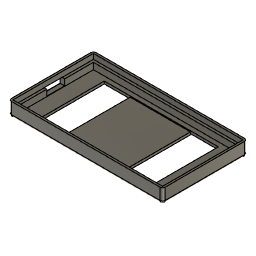
Caixa Sensores - Tampa (Autodesk Fusion 360 design; units mm, degrees)
Autodesk Fusion 360 part; units mm, degrees
note: some values were not read from the file. Set by a fixed rule: which face or edge a step refers to.
sketch "Esboço1" plane through (0, 0, 0) normal (0, 0, 1) x (1, 0, 0)
  line L0 (30, -16.5) -> (-30, -16.5)
  line L1 (-30, -16.5) -> (-30, 16.5)
  line L2 (-30, 16.5) -> (30, 16.5)
  line L3 (30, 16.5) -> (30, -16.5)
  line L4 (30, -16.5) -> (-30, 16.5) construction
  line L5 (-30, -16.5) -> (30, 16.5) construction
  dimension "d1" = 60
  dimension "d2" = 33
  constraint horizontal L0
  constraint perpendicular L0 L1
  constraint parallel L0 L2
  constraint parallel L1 L3
  constraint coincident L4 origin
  constraint coincident L5 origin
  measures "d1" distance of L1.end L2.end
  measures "d2" distance of L0.end L1.end
extrude "Extrusão1" add sketch "Esboço1" along normal blind 5.5
shell "Casca1" thickness 1.4 removed faces 1 at (10, 5.5, 5.5)
extrude "Extrusão2" add 1 faces at (28.6, -5.0333, 4.1333) along direction (-1, 0, 0) blind 0.4
extrude "Extrusão3" add 1 faces at (-9.6667, 15.1, 2.7667) along direction (0, -1, 0) blind 0.4
extrude "Extrusão4" add 1 faces at (-28.6, -5.1667, 4.1333) along direction (1, 0, 0) blind 0.4
extrude "Extrusão5" add 1 faces at (9.4, -15.1, 4.1333) along direction (0, 1, 0) blind 0.4
sketch "Esboço3" plane through (0, 0, 5.5) normal (0, 0, 1) x (-1, 0, 0)
  line L0 (-28.2, 14.7) -> (28.2, 14.7)
  line L1 (28.2, 14.7) -> (28.2, -14.7)
  line L2 (28.2, -14.7) -> (-28.2, -14.7)
  line L3 (-28.2, -14.7) -> (-28.2, 14.7)
  line L4 (-30, -16.5) -> (30, -16.5)
  line L5 (30, -16.5) -> (30, 16.5)
  line L6 (30, 16.5) -> (-30, 16.5)
  line L7 (-30, 16.5) -> (-30, -16.5)
  line L8 (29.2, -15.7) -> (-29.2, -15.7)
  line L9 (-29.2, -15.7) -> (-29.2, 15.7)
  line L10 (-29.2, 15.7) -> (29.2, 15.7)
  line L11 (29.2, 15.7) -> (29.2, -15.7)
  line L12 (29.2, -15.7) -> (-29.2, 15.7) construction
  line L13 (-29.2, -15.7) -> (29.2, 15.7) construction
  dimension "d16" = 60
  dimension "d17" = 33
  dimension "d18" = 58.4
  dimension "d19" = 31.4
  dimension "d48" = 60
  constraint horizontal L8
  constraint perpendicular L8 L9
  constraint parallel L8 L10
  constraint parallel L9 L11
  constraint coincident L12 origin
  constraint coincident L13 origin
  measures "d16" distance of L5.end L6.end
  measures "d17" distance of L4.end L5.end
  measures "d18" distance of L9.end L10.end
  measures "d19" distance of L8.end L9.end
  measures "d48" distance of L5.end L6.end
sketch "Esboço4" plane through (0, 0, 1.4) normal (0, 0, 1) x (-1, 0, 0)
  line L0 (28.2, 14.7) -> (-28.2, 14.7)
  line L1 (-28.2, 14.7) -> (-28.2, -14.7)
  line L2 (-28.2, -14.7) -> (28.2, -14.7)
  line L3 (28.2, -14.7) -> (28.2, 14.7)
  line L4 (-11.75, 13) -> (-22.25, 13)
  line L5 (-22.25, 13) -> (-22.25, -13)
  line L6 (-22.25, -13) -> (-11.75, -13)
  line L7 (-11.75, -13) -> (-11.75, 13)
  line L8 (-11.75, 13) -> (-22.25, -13) construction
  line L9 (-22.25, 13) -> (-11.75, -13) construction
  line L10 (22.25, 13) -> (11.75, 13)
  line L11 (11.75, 13) -> (11.75, -13)
  line L12 (11.75, -13) -> (22.25, -13)
  line L13 (22.25, -13) -> (22.25, 13)
  line L14 (22.25, 13) -> (11.75, -13) construction
  line L15 (11.75, 13) -> (22.25, -13) construction
  point P0 (-17, 0)
  point P1 (17, 0)
  dimension "d22" = 10.5
  dimension "d23" = 26
  dimension "d24" = 17
  dimension "d25" = 10.5
  dimension "d26" = 26
  constraint horizontal L4
  constraint perpendicular L4 L5
  constraint parallel L4 L6
  constraint parallel L5 L7
  constraint coincident L8 P0
  constraint coincident L9 P0
  constraint horizontal L10
  constraint perpendicular L10 L11
  constraint parallel L10 L12
  constraint parallel L11 L13
  constraint coincident L14 P1
  constraint coincident L15 P1
  measures "d22" distance of L5.end L6.end
  measures "d23" distance of L4.end L5.end
  measures "d24" distance of origin P1
  measures "d25" distance of L11.end L12.end
  measures "d26" distance of L10.end L11.end
extrude "Extrusão7" cut sketch "Esboço4" against normal blind 1 contours L4 L5 L6 L7 | L10 L11 L12 L13
sketch "Esboço5" plane through (-28.2, 0, 0) normal (1, 0, 0) x (0, 1, 0)
  line L0 (-14.7, 5.5) -> (-14.7, 1.4)
  line L1 (-14.7, 1.4) -> (14.7, 1.4)
  line L2 (14.7, 1.4) -> (14.7, 5.5)
  line L3 (14.7, 5.5) -> (-14.7, 5.5)
  line L4 (3.4905, 1.148) -> (-3.5095, 1.148)
  line L5 (-3.5095, 1.148) -> (-3.5095, 3.548)
  line L6 (-3.5095, 3.548) -> (3.4905, 3.548)
  line L7 (3.4905, 3.548) -> (3.4905, 1.148)
  line L8 (3.4905, 1.148) -> (-3.5095, 3.548) construction
  line L9 (-3.5095, 1.148) -> (3.4905, 3.548) construction
  point P0 (-0.0095, 2.348)
  dimension "d30" = 7
  dimension "d31" = 2.4
  constraint horizontal L4
  constraint perpendicular L4 L5
  constraint parallel L4 L6
  constraint parallel L5 L7
  constraint coincident L8 P0
  constraint coincident L9 P0
  measures "d30" distance of L5.end L6.end
  measures "d31" distance of L4.end L5.end
extrude "Extrusão8" cut sketch "Esboço5" against normal blind 5 contours L1 L5 L6 L7 | L1 L4 L5 L7
extrude "Extrusão11" cut sketch "Esboço3" against normal blind 2 contours L8 L9 L10 L11
extrude "Extrusão12" add 1 faces at (10, 5.5, 0) along direction (0, 0, -1) blind 0.6
extrude "Extrusão13" cut 1 faces at (10, 5.5, -0.6) along direction (0, 0, 1) blind 0.6
extrude "Extrusão14" cut 2 faces at (-15.25, -4.3333, 0.4) (18.75, -4.3333, 0.4) along direction (0, 0, -1) blind 3
extrude "Extrusão15" cut 1 faces at (-3.9167, 4.3333, 1.4) along direction (0, 0, -1) blind 0.4
sketch "Esboço6" plane through (0, 0, 1) normal (0, 0, 1) x (-1, 0, 0)
  line L0 (11.75, 13) -> (22.25, 13)
  line L1 (22.25, 13) -> (22.25, -13)
  line L2 (22.25, -13) -> (11.75, -13)
  line L3 (11.75, -13) -> (11.75, 13)
  line L4 (-22.25, 13) -> (-11.75, 13)
  line L5 (-11.75, 13) -> (-11.75, -13)
  line L6 (-11.75, -13) -> (-22.25, -13)
  line L7 (-22.25, -13) -> (-22.25, 13)
  line L8 (28.2, 14.7) -> (-28.2, 14.7)
  line L9 (-28.2, 14.7) -> (-28.2, -14.7)
  line L10 (-28.2, -14.7) -> (28.2, -14.7)
  line L11 (28.2, -14.7) -> (28.2, 14.7)
  line L12 (11.75, -13) -> (11.75, -12.6)
  line L13 (11.75, -13) -> (-11.75, -13)
  line L14 (11.75, -12.6) -> (-11.75, -12.6)
  line L15 (-11.75, -13) -> (-11.75, -12.6)
  dimension "d49" = 0.4
  constraint coincident L2.end L3.start
  constraint vertical L12
  constraint coincident L5.end L6.start
  constraint coincident L5 L14.end
  constraint perpendicular L5 L14
  measures "d49" distance of L2.end L12.end
extrude "Extrusão16" cut sketch "Esboço6" against normal blind 1 contours L3 L5 L12 L13 L14 L15
fillet "Arredondamento1" radius 1 2 edges at (30, 0, 0) (0, -16.5, 0)
fillet "Arredondamento2" radius 1 3 edges at (30, 16.5, 3.25) (29.7071, 16.5, 0.2929) (-0.5, 16.5, 0)
fillet "Arredondamento3" radius 1 2 edges at (29.7071, -16.2071, 0.2929) (30, -16.5, 3.25)
fillet "Arredondamento4" radius 1 5 edges at (-30, 16.5, 3.25) (-30, 16.2071, 0.2929) (-30, 0, 0) (-30, -16.2071, 0.2929) (-30, -16.5, 3.25)
